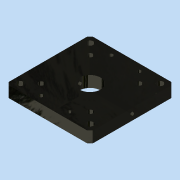
# Autodesk Inventor part: 00_XY_stage-CHUO_SEIKI_LD-647-R1-Top
Saved by Autodesk Inventor 2019.4 (Build 234330000, 330)
## iProperties
Created: 2019-05-02
Part Number: 00_XY_stage-CHUO_SEIKI_LD-647-R1-Top
Material: Generic
Document SubType Name: Modeling
Designer: diederichbenedict
Density: 1 g/cm^3
Appearance: Gunmetal
Mass: 26.0778 g
Surface Area: 101.151 cm^2
Volume: 26.0778 cm^3
Author: diederichbenedict
Autodesk Inventor part; units mm, degrees
ref_plane "YZ Plane" through (0, 0, 0) normal (1, 0, 0) x (0, 1, 0)
ref_plane "XZ Plane" through (0, 0, 0) normal (0, 1, 0) x (-1, 0, 0)
ref_plane "XY Plane" through (0, 0, 0) normal (0, 0, 1) x (1, 0, 0)
sketch "Sketch1" plane through (0, 0, 0) normal (0, 1, 0) x (-1, 0, 0)
  line L0 (-30, -30) -> (30, -30)
  line L1 (30, -30) -> (30, 30)
  line L2 (30, 30) -> (-30, 30)
  line L3 (-30, 30) -> (-30, -30)
  line L4 (-30, -30) -> (30, 30) construction
  line L5 (30, -30) -> (-30, 30) construction
  circle A0 centre (0, 0) radius 7.5
  circle A1 centre (-25, 25) radius 1.95 projected
  circle A2 centre (0, 25) radius 1.95 projected
  circle A3 centre (0, 25) radius 1.95 projected
  circle A4 centre (25, 0) radius 1.95 projected
  circle A5 centre (25, -25) radius 1.95 projected
  circle A6 centre (-25, 25) radius 1.95 projected
  circle A7 centre (-25, -25) radius 1.95 projected
  circle A8 centre (25, 25) radius 1.95 projected
  circle A9 centre (-25, 0) radius 1.95 projected
  circle A10 centre (0, -25) radius 1.95 projected
  line L6 (28, 30) -> (30, 28) projected
  line L7 (30, 28) -> (30, -28) projected
  line L8 (30, -28) -> (28, -30) projected
  line L9 (28, -30) -> (-28, -30) projected
  line L10 (-28, -30) -> (-30, -28) projected
  line L11 (-30, -28) -> (-30, 28) projected
  line L12 (-30, 28) -> (-28, 30) projected
  line L13 (-28, 30) -> (28, 30) projected
  dimension "d0" = 60
  dimension "d1" = 60
  dimension "d13" = 15
  constraints: 12 end point, 2 midpoint, 2 parallel, 1 centre point, 1 coincident, 1 horizontal, 1 perpendicular
  measures "d0" distance of L2.end L1.end
  measures "d1" distance of L1.end L0.end
  measures "d13" diameter of A0
extrude "Extrusion1" add sketch "Sketch1" along normal blind 8 contours L3 L10 L0 | L10 L3 L12 L2 L6 L1 L8 L0 | L8 L1 L0 | L3 L2 L12 | L6 L2 L1 | A1 | A2 | A4 | A5 | A7 | A8 | A9 | A10
sketch "Sketch2" plane through (0, 8, 0) normal (0, 1, 0) x (1, 0, 0)
  line L0 (30, 30) -> (-30, 30) projected
  line L1 (-30, 30) -> (-30, -30) projected
  line L2 (-30, -30) -> (30, -30) projected
  line L3 (30, -30) -> (30, 30) projected
  line L4 (17.5, -17.5) -> (-17.5, -17.5)
  line L5 (-17.5, -17.5) -> (-17.5, 17.5)
  line L6 (-17.5, 17.5) -> (17.5, 17.5)
  line L7 (17.5, 17.5) -> (17.5, -17.5)
  line L8 (17.5, -17.5) -> (-17.5, 17.5) construction
  line L9 (-17.5, -17.5) -> (17.5, 17.5) construction
  line L10 (0, -17.5) -> (0, 17.5)
  line L11 (-17.5, 0) -> (17.5, 0)
  point P0 (0, 0)
  dimension "d4" = 35
  dimension "d5" = 35
  constraints: 16 end point, 6 midpoint, 2 parallel, 1 horizontal, 1 perpendicular
  measures "d4" distance of L5.end L6.end
  measures "d5" distance of L4.end L5.end
hole "Hole1" at (-17.5, 8, 17.5) at (-17.5, 8, -17.5) at (17.5, 8, -17.5) at (17.5, 8, 17.5) direction (0, -1, 0) diameter 3.9 depth 10 tip angle 118
chamfer "Chamfer1" distance 2 angle 45 4 edges at (30, 4, 30) (30, 4, -30) (-30, 4, -30) (-30, 4, 30)
sketch "Sketch3" plane through (0, 8, 0) normal (0, 1, 0) x (1, 0, 0)
  line L0 (-28, -30) -> (-30, -28) projected
  line L1 (-28, -30) -> (28, -30) projected
  line L2 (30, -28) -> (28, -30) projected
  line L3 (30, -28) -> (30, 28) projected
  line L4 (28, 30) -> (30, 28) projected
  line L5 (28, 30) -> (-28, 30) projected
  line L6 (-30, 28) -> (-28, 30) projected
  line L7 (-30, 28) -> (-30, -28) projected
  circle A0 centre (17.5, 17.5) radius 1.95 projected
  circle A1 centre (-17.5, -17.5) radius 1.95 projected
  circle A2 centre (-17.5, 17.5) radius 1.95 projected
  circle A3 centre (17.5, -17.5) radius 1.95 projected
  circle A4 centre (0, 0) radius 7.5 projected
  line L8 (25, -25) -> (-25, -25)
  line L9 (-25, -25) -> (-25, 25)
  line L10 (-25, 25) -> (25, 25)
  line L11 (25, 25) -> (25, -25)
  line L12 (25, -25) -> (-25, 25) construction
  line L13 (-25, -25) -> (25, 25) construction
  dimension "d17" = 50
  dimension "d18" = 50
  constraints: 12 end point, 2 midpoint, 2 parallel, 1 horizontal, 1 perpendicular
  measures "d17" distance of L9.end L10.end
  measures "d18" distance of L8.end L9.end
hole "Hole2" at (-25, 8, -25) at (25, 8, -25) at (25, 8, 25) at (-25, 8, 25) direction (0, -1, 0) diameter 4.65 end through all
sketch "Sketch4" plane through (30, 0, 28) normal (1, 0, 0) x (0, 0, -1)
  line L0 (56, 8) -> (56, 0) projected
  line L1 (0, 8) -> (56, 8) projected
  line L2 (0, 0) -> (0, 8) projected
  line L3 (0, 0) -> (56, 0) projected
  circle A0 centre (28, 4) radius 1.5
  line L4 (-2, 8) -> (-2, 0) projected
  point P0 (28, 0)
  dimension "d26" = 3
  dimension "d27" = 4
  dimension "d28" = 30
  constraints: 1 centre point
  measures "d26" diameter of A0
  measures "d27" distance from line of A0.centre L1
  measures "d28" distance from line of A0.centre L4
extrude "Extrusion2" cut sketch "Sketch4" against normal through all contours A0
sketch "Sketch5" plane through (0, 8, 0) normal (0, 1, 0) x (1, 0, 0)
  circle A0 centre (25, -25) radius 2.325 projected
  circle A1 centre (-25, -25) radius 2.325 projected
  circle A2 centre (25, 25) radius 2.325 projected
  circle A3 centre (-25, 25) radius 2.325 projected
  circle A4 centre (10, -25) radius 1.45
  circle A5 centre (-10, -25) radius 1.45
  circle A6 centre (10, 25) radius 1.45
  circle A7 centre (-10, 25) radius 1.45
  point P0 (0, 0)
  dimension "d31" = 2.9
  dimension "d32" = 2.9
  dimension "d33" = 15
  dimension "d34" = 15
  dimension "d35" = 2.9
  dimension "d36" = 2.9
  constraints: 4 centre point
  measures "d31" diameter of A4
  measures "d32" diameter of A5
  measures "d33" distance of A4.centre A0.centre
  measures "d34" distance of A1.centre A5.centre
  measures "d35" diameter of A6
  measures "d36" diameter of A7
extrude "Extrusion3" cut sketch "Sketch5" against normal blind 10 contours A4 | A5 | A6 | A7
body "Solid1"
